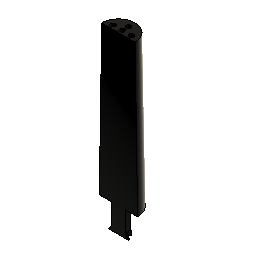
Balalaika assembly v16 (Autodesk Fusion 360 archive; units mm, degrees)
design "Neck 2"
Autodesk Fusion 360 part; units mm, degrees
note: some values were not read from the file. Chosen so that the rebuilt part matches the saved one: a side; which pieces of a blend or face edit are solid. Set by a fixed rule: which sketch regions a step uses.
sketch "Sketch1" plane through (0, 0, 0) normal (0, 0, 1) x (1, 0, 0)
  line L0 (-20, 0) -> (20, 0)
  circle A0 centre (0, 0) radius 20
  constraint horizontal L0
  constraint coincident A0.centre origin
  measures "d11" distance of L0.start
extrude "Extrude1" add sketch "Sketch1" along normal blind 157 contours L0 A0 picked at (5.5083, 3.7555)
chamfer "Chamfer1" distance 2.5 distance2 157 1 edges at (0, 20, 157) measured on face at (-8.2257, 18.2301, 52.3333)
sketch "Sketch2" plane through (0, 0, 0) normal (0, -1, 0) x (1, 0, 0)
  line L0 (20, 0) -> (17.5, 157)
  line L1 (17.5, 157) -> (-17.5, 157)
  line L2 (-17.5, 157) -> (-20, 0)
  line L3 (-20, 0) -> (20, 0)
  line L4 (0, 157) -> (-5, 157)
  line L5 (0, 157) -> (5, 157)
  line L6 (-5, 157) -> (-5, 145)
  line L7 (-5, 145) -> (-10, 140)
  line L8 (-10, 140) -> (10, 140)
  line L9 (10, 140) -> (5, 145)
  line L10 (5, 145) -> (5, 157)
  constraint midpoint L1 L4.start
  constraint coincident L1 L4.end
  constraint parallel L1 L4
  constraint coincident L1 L5.end
  constraint parallel L1 L5
  constraint perpendicular L1 L6
  constraint perpendicular L6 L8
  constraint perpendicular L7 L9
  constraint perpendicular L1 L10
extrude "Extrude2" cut sketch "Sketch2" against normal blind 7.5 contours L1 L4 L5 L6 L7 L8 L9 L10
sketch "Sketch3" plane through (0, 0, 0) normal (0, -1, 0) x (1, 0, 0)
  line L0 (-5, 145) -> (-5, 157)
  line L1 (-5, 157) -> (-17.5, 157)
  line L2 (-17.5, 157) -> (-20, 0)
  line L3 (-20, 0) -> (20, 0)
  line L4 (20, 0) -> (17.5, 157)
  line L5 (17.5, 157) -> (5, 157)
  line L6 (5, 157) -> (5, 145)
  line L7 (5, 145) -> (10, 140)
  line L8 (10, 140) -> (-10, 140)
  line L9 (-10, 140) -> (-5, 145)
  line L10 (-20, 0) -> (-7, 0)
  line L11 (20, 0) -> (7, 0)
  line L12 (-7, 0) -> (-7, -21)
  line L13 (7, 0) -> (7, -21)
  line L14 (-7, -21) -> (-7, -26)
  line L15 (-7, -21) -> (-10.3166, -26)
  line L16 (-10.3166, -26) -> (-7, -26)
  line L17 (7, -21) -> (10.3166, -26)
  line L18 (10.3166, -26) -> (-7, -26)
  dimension "d7" = 13
  dimension "d8" = 13
  dimension "d9" = 21
  dimension "d10" = 5
  dimension "d11" = 6
  dimension "d12" = 6
  constraint coincident L2.end L3.start
  constraint coincident L3 L10.end
  constraint coincident L3.end L4.start
  constraint coincident L3 L11.end
  constraint vertical L12
  constraint perpendicular L3 L13
  constraint parallel L12 L14
  constraint perpendicular L14 L16
  constraint perpendicular L13 L18
  measures "d7" distance of L2.end L10.end
  measures "d8" distance of L3.end L11.end
  measures "d9" distance of L10.end L12.end
  measures "d10" distance of L12.end L14.end
  measures "d11" distance of L12.end L15.end
  measures "d12" distance of L13.end L17.end
extrude "Extrude3" add sketch "Sketch3" against normal blind 6 contours L3 L12 L13 L14 L17 L18 | L14 L15 L16
sketch "Sketch4" plane through (0, 0, 0) normal (0, 0, -1) x (1, 0, 0)
  line L0 (-7, -6) -> (-7, 0)
  line L1 (-7, 0) -> (-20, 0)
  arc A0 (-20, 0) -> (20, 0) centre (0, 0) ccw
  line L2 (20, 0) -> (7, 0)
  line L3 (7, 0) -> (7, -6)
  line L4 (7, -6) -> (-7, -6)
sketch "Sketch5" plane through (0, 0, 0) normal (0, -1, 0) x (1, 0, 0)
  line L0 (-5, 145) -> (-5, 157)
  line L1 (-5, 157) -> (-17.5, 157)
  line L2 (-17.5, 157) -> (-20, 0)
  line L3 (-20, 0) -> (-7, 0)
  line L4 (-7, 0) -> (-7, -21)
  line L5 (-7, -21) -> (-10.3166, -26)
  line L6 (-10.3166, -26) -> (10.3166, -26)
  line L7 (10.3166, -26) -> (7, -21)
  line L8 (7, -21) -> (7, 0)
  line L9 (7, 0) -> (20, 0)
  line L10 (20, 0) -> (17.5, 157)
  line L11 (17.5, 157) -> (5, 157)
  line L12 (5, 157) -> (5, 145)
  line L13 (5, 145) -> (10, 140)
  line L14 (10, 140) -> (-10, 140)
  line L15 (-10, 140) -> (-5, 145)
  line L16 (-10, 140) -> (-5, 145)
  line L17 (-5, 145) -> (-5, 157)
  line L18 (-5, 157) -> (5, 157)
  line L19 (5, 157) -> (5, 145)
  line L20 (10, 140) -> (5, 145)
  line L21 (10, 140) -> (-10, 140)
  constraint coincident L14.end L15.start
  constraint coincident L0.start L15.end
  constraint coincident L0.end L1.start
  constraint coincident L11.end L12.start
  constraint coincident L12.end L13.start
  constraint coincident L13.end L14.start
extrude "Extrude4" add sketch "Sketch5" against normal blind 9 contours L0 L12 L13 L14 L15 L16 L17 L18 L19 L20 L21
sketch "Sketch6" plane through (0, 0, 157) normal (0, 0, 1) x (-1, 0, 0)
  line L0 (17.5, 0) -> (-17.5, 0)
  arc A0 (-17.5, 0) -> (17.5, 0) centre (0, 0) ccw
  line L1 (0, 0) -> (0, -4)
  circle A1 centre (0, -4) radius 2.5
  line L2 (0, -4) -> (9.5, -4)
  line L3 (0, -4) -> (-9.5, -4)
  circle A2 centre (-9.5, -4) radius 2.5
  circle A3 centre (9.5, -4) radius 2.5
  line L4 (0, -4) -> (0, -10.5)
  circle A4 centre (0, -10.5) radius 2.5
  dimension "d17" = 4
  dimension "d18" = 5
  dimension "d19" = 9.5
  dimension "d20" = 9.5
  dimension "d21" = 5
  dimension "d22" = 5
  dimension "d23" = 6.5
  dimension "d24" = 5
  constraint coincident A0.centre L1.start
  constraint perpendicular L0 L1
  constraint coincident L1.end A1.centre
  constraint perpendicular L1 L2
  constraint parallel L2 L3
  constraint coincident L3.end A2.centre
  constraint coincident L2.end A3.centre
  constraint perpendicular L2 L4
  constraint coincident L4.end A4.centre
  measures "d17" distance of A0.centre L1.end
  measures "d18" diameter of A1
  measures "d19" distance of L1.end L2.end
  measures "d20" distance of L1.end L3.end
  measures "d21" diameter of A2
  measures "d22" diameter of A3
  measures "d23" distance of L1.end L4.end
  measures "d24" diameter of A4
extrude "Extrude5" cut sketch "Sketch6" against normal blind 220 contours L1 A1 L2 | L1 A1 L3 | A1 L3 L4 | A1 L2 L4 | A2 | A3 | A4
sketch "Sketch7" plane through (0, 0, 0) normal (0, -1, 0) x (1, 0, 0)
  line L0 (17.5, 157) -> (-17.5, 157)
  line L1 (-17.5, 157) -> (-20, 0)
  line L2 (-20, 0) -> (-7, 0)
  line L3 (-7, 0) -> (-7, -21)
  line L4 (-7, -21) -> (-10.3166, -26)
  line L5 (-10.3166, -26) -> (10.3166, -26)
  line L6 (10.3166, -26) -> (7, -21)
  line L7 (7, -21) -> (7, 0)
  line L8 (7, 0) -> (20, 0)
  line L9 (20, 0) -> (17.5, 157)
sketch "Sketch8" plane through (0, 0, -26) normal (0, 0, -1) x (1, 0, 0)
  arc A0 (10.3166, -1.6371) -> (8, -6) centre (9.5, -4) ccw
  line L0 (10.3166, -1.6371) -> (10.3166, 0)
  line L1 (10.3166, 0) -> (-10.3166, 0)
  line L2 (-10.3166, 0) -> (-10.3166, -1.6371)
  arc A1 (-8, -6) -> (-10.3166, -1.6371) centre (-9.5, -4) ccw
  line L3 (-8, -6) -> (-1.5, -6)
  arc A2 (1.5, -6) -> (-1.5, -6) centre (0, -4) ccw
  line L4 (1.5, -6) -> (8, -6)
  line L5 (0, -4) -> (0, -10.5)
  constraint coincident A2.centre L5.start
  constraint vertical L5

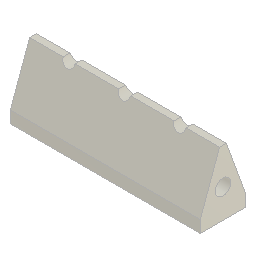
design "Bridge"
Autodesk Fusion 360 part; units mm, degrees
sketch "Sketch1" plane through (0, 0, 0) normal (0, 0, 1) x (1, 0, 0)
  line L0 (-20, 5) -> (20, 5)
  line L1 (20, 5) -> (20, -5)
  line L2 (20, -5) -> (-20, -5)
  line L3 (-20, -5) -> (-20, 5)
  line L4 (-20, 5) -> (20, -5) construction
  line L5 (20, 5) -> (-20, -5) construction
  line L6 (19.7, -4.7) -> (-19.7, -4.7)
  line L7 (-19.7, -4.7) -> (-19.7, 4.7)
  line L8 (-19.7, 4.7) -> (19.7, 4.7)
  line L9 (19.7, 4.7) -> (19.7, -4.7)
  dimension "d1" = 40
  dimension "d2" = 10
  dimension "d3" = 0.3
  constraint horizontal L0
  constraint perpendicular L0 L1
  constraint parallel L0 L2
  constraint parallel L1 L3
  constraint coincident L4 origin
  constraint coincident L5 origin
  measures "d1" distance of L1.end L2.end
  measures "d2" distance of L0.end L1.end
extrude "Extrude1" add sketch "Sketch1" along normal blind 11 contours L6 L7 L8 L9
sketch "Sketch2" plane through (19.7, 0, 0) normal (1, 0, 0) x (0, 1, 0)
  line L0 (-4.7, 0) -> (4.7, 0)
  line L1 (4.7, 0) -> (4.7, 11)
  line L2 (4.7, 11) -> (-4.7, 11)
  line L3 (-4.7, 11) -> (-4.7, 0)
  line L4 (0, 0) -> (-0.5801, 0) construction
  line L5 (0, 0) -> (0, 6) construction
  circle A0 centre (0, 6) radius 1.625
  dimension "d6" = 6
  dimension "d7" = 3.25
  constraint coincident L4.start L5.start
  constraint coincident L0 L4.end
  constraint perpendicular L4 L5
  constraint coincident L5.end A0.centre
  measures "d6" distance of L4.start L5.end
  measures "d7" diameter of A0
extrude "Extrude2" add 1 faces at (6.5667, -1.5667, 11) along direction (0, 0, 1) blind 2.5
sketch "Sketch3" plane through (0, -4.7, 0) normal (0, -1, 0) x (1, 0, 0)
  line L0 (-19.7, 0) -> (19.7, 0)
  line L1 (19.7, 0) -> (19.7, 13.5)
  line L2 (19.7, 13.5) -> (-19.7, 13.5)
  line L3 (-19.7, 13.5) -> (-19.7, 0)
  circle A0 centre (0, 13.5) radius 1.25
  line L4 (1.25, 13.5) -> (10.25, 13.5) construction
  line L5 (10.25, 13.5) -> (12.75, 13.5) construction
  circle A1 centre (11.5, 13.5) radius 1.25
  line L6 (0, 14.75) -> (0, 12.25) construction
  circle A2 centre (-11.5, 13.5) radius 1.25
  dimension "d11" = 9
  dimension "d12" = 2.5
  constraint midpoint L2 A0.centre
  constraint coincident A0 L4.start
  constraint coincident L2 L4.start
  constraint coincident L2 L4.end
  constraint parallel L2 L5
  constraint midpoint L5 A1.centre
  constraint coincident L5.end A1
  constraint coincident A0 L6.start
  constraint coincident A0 L6.end
  constraint perpendicular L2 L6
  constraint symmetric A1 L6 A2
  measures "d11" distance of L4.start L4.end
  measures "d12" distance of L4.end L5.end
extrude "Extrude3" cut sketch "Sketch3" against normal blind 25 contours L2 A2 | L2 A1 | L2 A0 picked at (-11.7825, 12.8706) picked at (11.2175, 12.8706) picked at (-0.3939, 13.1964)
extrude "Extrude4" add sketch "Sketch3" against normal blind 9.4 contours L2 A2 | L2 A1 | L2 A0 picked at (-11.7825, 12.8706) picked at (11.2175, 12.8706) picked at (-0.3939, 13.1964)
chamfer "Chamfer1" distance 4 distance2 11 2 edges at (0, -4.7, 13.5) (0, 4.7, 13.5) measured on face at (6.5667, -1.5667, 13.5) measured on face at (6.5667, -1.5667, 13.5)
extrude "Extrude5" cut sketch "Sketch2" against normal blind 74 contours A0
extrude "Extrude6" cut sketch "Sketch3" against normal blind 12 contours L2 A2 | L2 A1 | L2 A0 picked at (-11.7825, 12.8706) picked at (11.2175, 12.8706) picked at (-0.3939, 13.1964)
equation "d4 = 9.5 mm + 1.5 mm"
equation "d18 = 13.5 mm - 2.5 mm"
